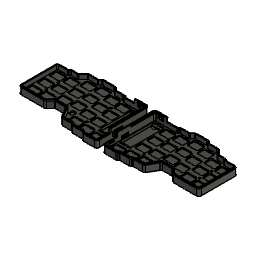
mriya-classic-fdm-301645-v1.00 (Autodesk Fusion 360 design; units mm, degrees)
Autodesk Fusion 360 part; units mm, degrees
(part 1 of 2)
sketch "mriya-classic-fdm-301645" plane through (0, 0, 0) normal (0, 0, 1) x (1, 0, 0)
  line L0 (-101.0213, 15.6719) -> (-94.7787, 21.9145) construction
  line L1 (-26.4858, 1.079) -> (-27.6142, 2.2074) construction
  line L2 (-138.1, 14.7932) -> (-103.1426, 14.7932) construction
  line L3 (-44.0716, 2.7932) -> (-29.0284, 2.7932) construction
  line L4 (-8.6, 0.4932) -> (-25.0716, 0.4932) construction
  line L5 (-64.4741, 6.1094) -> (-72.7517, 20.7608) construction
  line L6 (-45.4858, 3.379) -> (-46.6142, 4.5074) construction
  line L7 (-122.6142, 71.579) -> (-121.4858, 72.7074) construction
  line L8 (-101.0716, 81.2932) -> (-87.2284, 81.2932) construction
  line L9 (-138.1, 70.9932) -> (-124.0284, 70.9932) construction
  line L10 (-92.6574, 22.7932) -> (-76.2344, 22.7932) construction
  line L11 (-48.0284, 5.0932) -> (-62.7328, 5.0932) construction
  line L12 (-82.0716, 84.7932) -> (-64.7284, 84.7932) construction
  line L13 (-58.5716, 80.2932) -> (-45.7284, 80.2932) construction
  line L14 (-24.1, 19.4932) -> (-7.1, 19.4932) construction
  line L15 (-25.6, 20.9932) -> (-25.6, 77.9932) construction
  line L16 (-83.4858, 84.2074) -> (-85.8142, 81.879) construction
  line L17 (-63.3142, 84.2074) -> (-59.9858, 80.879) construction
  line L18 (-139.6, 69.4932) -> (-139.6, 16.2932) construction
  line L19 (-43.1858, 78.579) -> (-44.3142, 79.7074) construction
  line L20 (-99.4, 40.3932) -> (-99.4, 27.9932) construction
  line L21 (-98.6, 41.1932) -> (-86.2, 41.1932) construction
  line L22 (-98.6, 27.1932) -> (-86.2, 27.1932) construction
  line L23 (-85.4, 40.3932) -> (-85.4, 27.9932) construction
  line L24 (-42.4, 56.0932) -> (-42.4, 43.6932) construction
  line L25 (-41.6, 56.8932) -> (-29.2, 56.8932) construction
  line L26 (-41.6, 42.8932) -> (-29.2, 42.8932) construction
  line L27 (-28.4, 56.0932) -> (-28.4, 43.6932) construction
  line L28 (-61.4, 58.3932) -> (-61.4, 45.9932) construction
  line L29 (-60.6, 59.1932) -> (-48.2, 59.1932) construction
  line L30 (-60.6, 45.1932) -> (-48.2, 45.1932) construction
  line L31 (-47.4, 58.3932) -> (-47.4, 45.9932) construction
  line L32 (-137.4, 68.0932) -> (-137.4, 55.6932) construction
  line L33 (-136.6, 68.8932) -> (-124.2, 68.8932) construction
  line L34 (-136.6, 54.8932) -> (-124.2, 54.8932) construction
  line L35 (-123.4, 68.0932) -> (-123.4, 55.6932) construction
  line L36 (-61.4, 39.3932) -> (-61.4, 26.9932) construction
  line L37 (-60.6, 40.1932) -> (-48.2, 40.1932) construction
  line L38 (-60.6, 26.1932) -> (-48.2, 26.1932) construction
  line L39 (-47.4, 39.3932) -> (-47.4, 26.9932) construction
  line L40 (-42.4, 18.0932) -> (-42.4, 5.6932) construction
  line L41 (-41.6, 18.8932) -> (-29.2, 18.8932) construction
  line L42 (-41.6, 4.8932) -> (-29.2, 4.8932) construction
  line L43 (-28.4, 18.0932) -> (-28.4, 5.6932) construction
  line L44 (-23.4, 15.7932) -> (-23.4, 3.3932) construction
  line L45 (-22.6, 16.5932) -> (-10.2, 16.5932) construction
  line L46 (-22.6, 2.5932) -> (-10.2, 2.5932) construction
  line L47 (-9.4, 15.7932) -> (-9.4, 3.3932) construction
  line L48 (-137.4, 49.0932) -> (-137.4, 36.6932) construction
  line L49 (-136.6, 49.8932) -> (-124.2, 49.8932) construction
  line L50 (-136.6, 35.8932) -> (-124.2, 35.8932) construction
  line L51 (-123.4, 49.0932) -> (-123.4, 36.6932) construction
  line L52 (-118.4, 51.3932) -> (-118.4, 38.9932) construction
  line L53 (-117.6, 52.1932) -> (-105.2, 52.1932) construction
  line L54 (-117.6, 38.1932) -> (-105.2, 38.1932) construction
  line L55 (-104.4, 51.3932) -> (-104.4, 38.9932) construction
  line L56 (-137.4, 30.0932) -> (-137.4, 17.6932) construction
  line L57 (-136.6, 30.8932) -> (-124.2, 30.8932) construction
  line L58 (-136.6, 16.8932) -> (-124.2, 16.8932) construction
  line L59 (-123.4, 30.0932) -> (-123.4, 17.6932) construction
  line L60 (-61.4, 20.3932) -> (-61.4, 7.9932) construction
  line L61 (-60.6, 21.1932) -> (-48.2, 21.1932) construction
  line L62 (-60.6, 7.1932) -> (-48.2, 7.1932) construction
  line L63 (-47.4, 20.3932) -> (-47.4, 7.9932) construction
  line L64 (-80.4, 43.8932) -> (-80.4, 31.4932) construction
  line L65 (-79.6, 44.6932) -> (-67.2, 44.6932) construction
  line L66 (-79.6, 30.6932) -> (-67.2, 30.6932) construction
  line L67 (-66.4, 43.8932) -> (-66.4, 31.4932) construction
  line L68 (-80.4, 81.8932) -> (-80.4, 69.4932) construction
  line L69 (-79.6, 82.6932) -> (-67.2, 82.6932) construction
  line L70 (-79.6, 68.6932) -> (-67.2, 68.6932) construction
  line L71 (-66.4, 81.8932) -> (-66.4, 69.4932) construction
  line L72 (-42.4, 37.0932) -> (-42.4, 24.6932) construction
  line L73 (-41.6, 37.8932) -> (-29.2, 37.8932) construction
  line L74 (-41.6, 23.8932) -> (-29.2, 23.8932) construction
  line L75 (-28.4, 37.0932) -> (-28.4, 24.6932) construction
  line L76 (-118.4, 32.3932) -> (-118.4, 19.9932) construction
  line L77 (-117.6, 33.1932) -> (-105.2, 33.1932) construction
  line L78 (-117.6, 19.1932) -> (-105.2, 19.1932) construction
  line L79 (-104.4, 32.3932) -> (-104.4, 19.9932) construction
  line L80 (-61.4, 77.3932) -> (-61.4, 64.9932) construction
  line L81 (-60.6, 78.1932) -> (-48.2, 78.1932) construction
  line L82 (-60.6, 64.1932) -> (-48.2, 64.1932) construction
  line L83 (-47.4, 77.3932) -> (-47.4, 64.9932) construction
  line L84 (-42.4, 75.0932) -> (-42.4, 62.6932) construction
  line L85 (-41.6, 75.8932) -> (-29.2, 75.8932) construction
  line L86 (-41.6, 61.8932) -> (-29.2, 61.8932) construction
  line L87 (-28.4, 75.0932) -> (-28.4, 62.6932) construction
  line L88 (-118.4, 70.3932) -> (-118.4, 57.9932) construction
  line L89 (-117.6, 71.1932) -> (-105.2, 71.1932) construction
  line L90 (-117.6, 57.1932) -> (-105.2, 57.1932) construction
  line L91 (-104.4, 70.3932) -> (-104.4, 57.9932) construction
  line L92 (-99.4, 59.3932) -> (-99.4, 46.9932) construction
  line L93 (-98.6, 60.1932) -> (-86.2, 60.1932) construction
  line L94 (-98.6, 46.1932) -> (-86.2, 46.1932) construction
  line L95 (-85.4, 59.3932) -> (-85.4, 46.9932) construction
  line L96 (-80.4, 62.8932) -> (-80.4, 50.4932) construction
  line L97 (-79.6, 63.6932) -> (-67.2, 63.6932) construction
  line L98 (-79.6, 49.6932) -> (-67.2, 49.6932) construction
  line L99 (-66.4, 62.8932) -> (-66.4, 50.4932) construction
  line L100 (-99.4, 78.3932) -> (-99.4, 65.9932) construction
  line L101 (-98.6, 79.1932) -> (-86.2, 79.1932) construction
  line L102 (-98.6, 65.1932) -> (-86.2, 65.1932) construction
  line L103 (-85.4, 78.3932) -> (-85.4, 65.9932) construction
  circle A0 centre (-120.9, 53.5432) radius 1.7
  circle A1 centre (-120.9, 34.5432) radius 1.7
  circle A2 centre (-68.3, 23.4932) radius 4
  circle A3 centre (-44.9, 22.5432) radius 1.7
  circle A4 centre (-44.9, 60.5432) radius 1.7
  arc A5 (-43.1858, 78.579) -> (-41.7716, 77.9932) centre (-41.7716, 79.9932) ccw construction
  arc A6 (-44.3142, 79.7074) -> (-45.7284, 80.2932) centre (-45.7285, 78.2931) ccw construction
  arc A7 (-59.9858, 80.879) -> (-58.5716, 80.2932) centre (-58.5716, 82.2931) ccw construction
  arc A8 (-63.3142, 84.2074) -> (-64.7284, 84.7932) centre (-64.7285, 82.7931) ccw construction
  arc A9 (-82.0716, 84.7932) -> (-83.4858, 84.2074) centre (-82.0716, 82.7933) ccw construction
  arc A10 (-87.2284, 81.2932) -> (-85.8142, 81.879) centre (-87.2284, 83.2932) ccw construction
  arc A11 (-101.0716, 81.2932) -> (-102.4858, 80.7074) centre (-101.0716, 79.2933) ccw construction
  arc A12 (-120.0716, 73.2932) -> (-121.4858, 72.7074) centre (-120.0716, 71.2933) ccw construction
  arc A13 (-124.0284, 70.9932) -> (-122.6142, 71.579) centre (-124.0284, 72.9932) ccw construction
  arc A14 (-138.1, 70.9932) -> (-139.6, 69.4932) centre (-138.1, 69.4932) ccw construction
  arc A15 (-139.6, 16.2932) -> (-138.1, 14.7932) centre (-138.1, 16.2932) ccw construction
  arc A16 (-103.1426, 14.7932) -> (-101.0213, 15.6719) centre (-103.1426, 17.7931) ccw construction
  arc A17 (-92.6574, 22.7932) -> (-94.7787, 21.9145) centre (-92.6573, 19.7931) ccw construction
  arc A18 (-72.7517, 20.7608) -> (-76.2344, 22.7932) centre (-76.2344, 18.793) ccw construction
  arc A19 (-64.4741, 6.1094) -> (-62.7328, 5.0932) centre (-62.7328, 7.0932) ccw construction
  arc A20 (-46.6142, 4.5074) -> (-48.0284, 5.0932) centre (-48.0284, 3.0933) ccw construction
  arc A21 (-45.4858, 3.379) -> (-44.0716, 2.7932) centre (-44.0715, 4.7933) ccw construction
  arc A22 (-27.6142, 2.2074) -> (-29.0284, 2.7932) centre (-29.0284, 0.7933) ccw construction
  arc A23 (-26.4858, 1.079) -> (-25.0716, 0.4932) centre (-25.0715, 2.4933) ccw construction
  arc A24 (-8.6, 0.4932) -> (-7.1, 1.9932) centre (-8.6, 1.9932) ccw construction
  arc A25 (-25.6, 20.9932) -> (-24.1, 19.4932) centre (-24.1, 20.9932) ccw construction
  line L104 (-7.1, 1.9932) -> (-7.1, 76.4932) construction
  line L105 (-41.7716, 77.9932) -> (-8.6, 77.9932) construction
  arc A26 (-7.1, 76.4932) -> (-8.6, 77.9932) centre (-8.6, 76.4932) ccw construction
  arc A27 (-136.6, 68.8932) -> (-137.4, 68.0932) centre (-136.6, 68.0932) ccw construction
  arc A28 (-123.4, 68.0932) -> (-124.2, 68.8932) centre (-124.2, 68.0932) ccw construction
  arc A29 (-124.2, 54.8932) -> (-123.4, 55.6932) centre (-124.2, 55.6932) ccw construction
  arc A30 (-137.4, 55.6932) -> (-136.6, 54.8932) centre (-136.6, 55.6932) ccw construction
  arc A31 (-136.6, 49.8932) -> (-137.4, 49.0932) centre (-136.6, 49.0932) ccw construction
  arc A32 (-123.4, 49.0932) -> (-124.2, 49.8932) centre (-124.2, 49.0932) ccw construction
  arc A33 (-124.2, 35.8932) -> (-123.4, 36.6932) centre (-124.2, 36.6932) ccw construction
  arc A34 (-137.4, 36.6932) -> (-136.6, 35.8932) centre (-136.6, 36.6932) ccw construction
  arc A35 (-136.6, 30.8932) -> (-137.4, 30.0932) centre (-136.6, 30.0932) ccw construction
  arc A36 (-123.4, 30.0932) -> (-124.2, 30.8932) centre (-124.2, 30.0932) ccw construction
  arc A37 (-124.2, 16.8932) -> (-123.4, 17.6932) centre (-124.2, 17.6932) ccw construction
  arc A38 (-137.4, 17.6932) -> (-136.6, 16.8932) centre (-136.6, 17.6932) ccw construction
  arc A39 (-118.4, 19.9932) -> (-117.6, 19.1932) centre (-117.6, 19.9932) ccw construction
  arc A40 (-105.2, 19.1932) -> (-104.4, 19.9932) centre (-105.2, 19.9932) ccw construction
  arc A41 (-104.4, 32.3932) -> (-105.2, 33.1932) centre (-105.2, 32.3932) ccw construction
  arc A42 (-117.6, 33.1932) -> (-118.4, 32.3932) centre (-117.6, 32.3932) ccw construction
  arc A43 (-105.2, 38.1932) -> (-104.4, 38.9932) centre (-105.2, 38.9932) ccw construction
  arc A44 (-118.4, 38.9932) -> (-117.6, 38.1932) centre (-117.6, 38.9932) ccw construction
  arc A45 (-117.6, 52.1932) -> (-118.4, 51.3932) centre (-117.6, 51.3932) ccw construction
  arc A46 (-104.4, 51.3932) -> (-105.2, 52.1932) centre (-105.2, 51.3932) ccw construction
  arc A47 (-118.4, 57.9932) -> (-117.6, 57.1932) centre (-117.6, 57.9932) ccw construction
  arc A48 (-105.2, 57.1932) -> (-104.4, 57.9932) centre (-105.2, 57.9932) ccw construction
  arc A49 (-104.4, 70.3932) -> (-105.2, 71.1932) centre (-105.2, 70.3932) ccw construction
  arc A50 (-117.6, 71.1932) -> (-118.4, 70.3932) centre (-117.6, 70.3932) ccw construction
  arc A51 (-98.6, 79.1932) -> (-99.4, 78.3932) centre (-98.6, 78.3932) ccw construction
  arc A52 (-85.4, 78.3932) -> (-86.2, 79.1932) centre (-86.2, 78.3932) ccw construction
  arc A53 (-86.2, 65.1932) -> (-85.4, 65.9932) centre (-86.2, 65.9932) ccw construction
  arc A54 (-99.4, 65.9932) -> (-98.6, 65.1932) centre (-98.6, 65.9932) ccw construction
  arc A55 (-98.6, 60.1932) -> (-99.4, 59.3932) centre (-98.6, 59.3932) ccw construction
  arc A56 (-85.4, 59.3932) -> (-86.2, 60.1932) centre (-86.2, 59.3932) ccw construction
  arc A57 (-86.2, 46.1932) -> (-85.4, 46.9932) centre (-86.2, 46.9932) ccw construction
  arc A58 (-99.4, 46.9932) -> (-98.6, 46.1932) centre (-98.6, 46.9932) ccw construction
  arc A59 (-98.6, 41.1932) -> (-99.4, 40.3932) centre (-98.6, 40.3932) ccw construction
  arc A60 (-99.4, 27.9932) -> (-98.6, 27.1932) centre (-98.6, 27.9932) ccw construction
  arc A61 (-86.2, 27.1932) -> (-85.4, 27.9932) centre (-86.2, 27.9932) ccw construction
  arc A62 (-85.4, 40.3932) -> (-86.2, 41.1932) centre (-86.2, 40.3932) ccw construction
  arc A63 (-80.4, 31.4932) -> (-79.6, 30.6932) centre (-79.6, 31.4932) ccw construction
  arc A64 (-79.6, 44.6932) -> (-80.4, 43.8932) centre (-79.6, 43.8932) ccw construction
  arc A65 (-66.4, 43.8932) -> (-67.2, 44.6932) centre (-67.2, 43.8932) ccw construction
  arc A66 (-67.2, 30.6932) -> (-66.4, 31.4932) centre (-67.2, 31.4932) ccw construction
  arc A67 (-67.2, 49.6932) -> (-66.4, 50.4932) centre (-67.2, 50.4932) ccw construction
  arc A68 (-80.4, 50.4932) -> (-79.6, 49.6932) centre (-79.6, 50.4932) ccw construction
  arc A69 (-79.6, 63.6932) -> (-80.4, 62.8932) centre (-79.6, 62.8932) ccw construction
  arc A70 (-66.4, 62.8932) -> (-67.2, 63.6932) centre (-67.2, 62.8932) ccw construction
  arc A71 (-67.2, 68.6932) -> (-66.4, 69.4932) centre (-67.2, 69.4932) ccw construction
  arc A72 (-80.4, 69.4932) -> (-79.6, 68.6932) centre (-79.6, 69.4932) ccw construction
  arc A73 (-79.6, 82.6932) -> (-80.4, 81.8932) centre (-79.6, 81.8932) ccw construction
  arc A74 (-66.4, 81.8932) -> (-67.2, 82.6932) centre (-67.2, 81.8932) ccw construction
  arc A75 (-60.6, 78.1932) -> (-61.4, 77.3932) centre (-60.6, 77.3932) ccw construction
  arc A76 (-61.4, 64.9932) -> (-60.6, 64.1932) centre (-60.6, 64.9932) ccw construction
  arc A77 (-48.2, 64.1932) -> (-47.4, 64.9932) centre (-48.2, 64.9932) ccw construction
  arc A78 (-47.4, 77.3932) -> (-48.2, 78.1932) centre (-48.2, 77.3932) ccw construction
  arc A79 (-47.4, 58.3932) -> (-48.2, 59.1932) centre (-48.2, 58.3932) ccw construction
  arc A80 (-60.6, 59.1932) -> (-61.4, 58.3932) centre (-60.6, 58.3932) ccw construction
  arc A81 (-61.4, 45.9932) -> (-60.6, 45.1932) centre (-60.6, 45.9932) ccw construction
  arc A82 (-48.2, 45.1932) -> (-47.4, 45.9932) centre (-48.2, 45.9932) ccw construction
  arc A83 (-47.4, 39.3932) -> (-48.2, 40.1932) centre (-48.2, 39.3932) ccw construction
  arc A84 (-60.6, 40.1932) -> (-61.4, 39.3932) centre (-60.6, 39.3932) ccw construction
  arc A85 (-61.4, 26.9932) -> (-60.6, 26.1932) centre (-60.6, 26.9932) ccw construction
  arc A86 (-48.2, 26.1932) -> (-47.4, 26.9932) centre (-48.2, 26.9932) ccw construction
  arc A87 (-47.4, 20.3932) -> (-48.2, 21.1932) centre (-48.2, 20.3932) ccw construction
  arc A88 (-60.6, 21.1932) -> (-61.4, 20.3932) centre (-60.6, 20.3932) ccw construction
  arc A89 (-61.4, 7.9932) -> (-60.6, 7.1932) centre (-60.6, 7.9932) ccw construction
  arc A90 (-48.2, 7.1932) -> (-47.4, 7.9932) centre (-48.2, 7.9932) ccw construction
  arc A91 (-42.4, 5.6932) -> (-41.6, 4.8932) centre (-41.6, 5.6932) ccw construction
  arc A92 (-29.2, 4.8932) -> (-28.4, 5.6932) centre (-29.2, 5.6932) ccw construction
  arc A93 (-28.4, 18.0932) -> (-29.2, 18.8932) centre (-29.2, 18.0932) ccw construction
  arc A94 (-41.6, 18.8932) -> (-42.4, 18.0932) centre (-41.6, 18.0932) ccw construction
  arc A95 (-23.4, 3.3932) -> (-22.6, 2.5932) centre (-22.6, 3.3932) ccw construction
  arc A96 (-10.2, 2.5932) -> (-9.4, 3.3932) centre (-10.2, 3.3932) ccw construction
  arc A97 (-9.4, 15.7932) -> (-10.2, 16.5932) centre (-10.2, 15.7932) ccw construction
  arc A98 (-22.6, 16.5932) -> (-23.4, 15.7932) centre (-22.6, 15.7932) ccw construction
  arc A99 (-29.2, 23.8932) -> (-28.4, 24.6932) centre (-29.2, 24.6932) ccw construction
  arc A100 (-42.4, 24.6932) -> (-41.6, 23.8932) centre (-41.6, 24.6932) ccw construction
  arc A101 (-41.6, 37.8932) -> (-42.4, 37.0932) centre (-41.6, 37.0932) ccw construction
  arc A102 (-28.4, 37.0932) -> (-29.2, 37.8932) centre (-29.2, 37.0932) ccw construction
  arc A103 (-29.2, 42.8932) -> (-28.4, 43.6932) centre (-29.2, 43.6932) ccw construction
  arc A104 (-42.4, 43.6932) -> (-41.6, 42.8932) centre (-41.6, 43.6932) ccw construction
  arc A105 (-41.6, 56.8932) -> (-42.4, 56.0932) centre (-41.6, 56.0932) ccw construction
  arc A106 (-28.4, 56.0932) -> (-29.2, 56.8932) centre (-29.2, 56.0932) ccw construction
  arc A107 (-29.2, 61.8932) -> (-28.4, 62.6932) centre (-29.2, 62.6932) ccw construction
  arc A108 (-42.4, 62.6932) -> (-41.6, 61.8932) centre (-41.6, 62.6932) ccw construction
  arc A109 (-41.6, 75.8932) -> (-42.4, 75.0932) centre (-41.6, 75.0932) ccw construction
  arc A110 (-28.4, 75.0932) -> (-29.2, 75.8932) centre (-29.2, 75.0932) ccw construction
  circle A111 centre (-22.6, 22.4932) radius 1.15
  circle A112 centre (-10.1, 22.4932) radius 1.15
  line L106 (-102.4858, 80.7074) -> (-109.0213, 74.1719) construction
  line L107 (-120.0716, 73.2932) -> (-111.1426, 73.2932) construction
  arc A113 (-111.1426, 73.2932) -> (-109.0213, 74.1719) centre (-111.1426, 76.2932) ccw construction
  arc A114 (-64.7284, 82.7932) -> (-64.7285, 82.7932) centre (-64.7285, 82.7931) ccw
  arc A115 (-45.7284, 78.2932) -> (-45.7285, 78.2932) centre (-45.7285, 78.2931) ccw
  arc A116 (-25.0716, 2.4932) -> (-25.0715, 2.4932) centre (-25.0715, 2.4933) ccw
  arc A117 (-44.0716, 4.7932) -> (-44.0715, 4.7932) centre (-44.0715, 4.7933) ccw
  line L108 (-138.9, 58.3932) -> (-138.9, 66.8932)
  line L109 (-136.9, 68.8932) -> (-123.9, 68.8932)
  arc A118 (-121.9, 66.8932) -> (-123.9, 68.8932) centre (-123.9, 66.8932) ccw
  arc A119 (-138.9, 58.3932) -> (-136.9, 56.3932) centre (-136.9, 58.3932) ccw
  arc A120 (-136.9, 68.8932) -> (-138.9, 66.8932) centre (-136.9, 66.8932) ccw
  arc A121 (-138.9, 39.3932) -> (-136.9, 37.3932) centre (-136.9, 39.3932) ccw
  line L110 (-138.9, 39.3932) -> (-138.9, 47.8932)
  arc A122 (-136.9, 49.8932) -> (-138.9, 47.8932) centre (-136.9, 47.8932) ccw
  line L111 (-136.9, 49.8932) -> (-123.9, 49.8932)
  arc A123 (-121.9, 47.8932) -> (-123.9, 49.8932) centre (-123.9, 47.8932) ccw
  arc A124 (-123.9, 18.3932) -> (-121.9, 20.3932) centre (-123.9, 20.3932) ccw
  line L112 (-123.9, 18.3932) -> (-136.9, 18.3932)
  arc A125 (-138.9, 20.3932) -> (-136.9, 18.3932) centre (-136.9, 20.3932) ccw
  line L113 (-138.9, 20.3932) -> (-138.9, 28.8932)
  arc A126 (-136.9, 30.8932) -> (-138.9, 28.8932) centre (-136.9, 28.8932) ccw
  line L114 (-136.9, 30.8932) -> (-123.9, 30.8932)
  arc A127 (-121.9, 28.8932) -> (-123.9, 30.8932) centre (-123.9, 28.8932) ccw
  line L115 (-121.9, 28.8932) -> (-121.9, 20.3932)
  arc A128 (-104.9, 58.6932) -> (-102.9, 60.6932) centre (-104.9, 60.6932) ccw
  line L116 (-104.9, 58.6932) -> (-117.9, 58.6932)
  arc A129 (-119.9, 60.6932) -> (-117.9, 58.6932) centre (-117.9, 60.6932) ccw
  line L117 (-119.9, 60.6932) -> (-119.9, 69.1932)
  arc A130 (-117.9, 71.1932) -> (-119.9, 69.1932) centre (-117.9, 69.1932) ccw
  line L118 (-117.9, 71.1932) -> (-104.9, 71.1932)
  arc A131 (-102.9, 69.1932) -> (-104.9, 71.1932) centre (-104.9, 69.1932) ccw
  line L119 (-102.9, 69.1932) -> (-102.9, 60.6932)
  arc A132 (-104.9, 39.6932) -> (-102.9, 41.6932) centre (-104.9, 41.6932) ccw
  line L120 (-104.9, 39.6932) -> (-117.9, 39.6932)
  arc A133 (-119.9, 41.6932) -> (-117.9, 39.6932) centre (-117.9, 41.6932) ccw
  arc A134 (-102.9, 50.1932) -> (-104.9, 52.1932) centre (-104.9, 50.1932) ccw
  line L121 (-102.9, 50.1932) -> (-102.9, 41.6932)
  arc A135 (-104.9, 20.6932) -> (-102.9, 22.6932) centre (-104.9, 22.6932) ccw
  line L122 (-104.9, 20.6932) -> (-117.9, 20.6932)
  arc A136 (-119.9, 22.6932) -> (-117.9, 20.6932) centre (-117.9, 22.6932) ccw
  arc A137 (-102.9, 31.1932) -> (-104.9, 33.1932) centre (-104.9, 31.1932) ccw
  line L123 (-102.9, 31.1932) -> (-102.9, 22.6932)
  arc A138 (-85.9, 66.6932) -> (-83.9, 68.6932) centre (-85.9, 68.6932) ccw
  line L124 (-85.9, 66.6932) -> (-98.9, 66.6932)
  arc A139 (-100.9, 68.6932) -> (-98.9, 66.6932) centre (-98.9, 68.6932) ccw
  line L125 (-100.9, 68.6932) -> (-100.9, 77.1932)
  arc A140 (-98.9, 79.1932) -> (-100.9, 77.1932) centre (-98.9, 77.1932) ccw
  line L126 (-98.9, 79.1932) -> (-85.9, 79.1932)
  arc A141 (-83.9, 77.1932) -> (-85.9, 79.1932) centre (-85.9, 77.1932) ccw
  line L127 (-83.9, 77.1932) -> (-83.9, 68.6932)
  arc A142 (-85.9, 47.6932) -> (-83.9, 49.6932) centre (-85.9, 49.6932) ccw
  line L128 (-85.9, 47.6932) -> (-98.9, 47.6932)
  arc A143 (-100.9, 49.6932) -> (-98.9, 47.6932) centre (-98.9, 49.6932) ccw
  line L129 (-100.9, 49.6932) -> (-100.9, 58.1932)
  arc A144 (-98.9, 60.1932) -> (-100.9, 58.1932) centre (-98.9, 58.1932) ccw
  line L130 (-98.9, 60.1932) -> (-85.9, 60.1932)
  arc A145 (-83.9, 58.1932) -> (-85.9, 60.1932) centre (-85.9, 58.1932) ccw
  line L131 (-83.9, 58.1932) -> (-83.9, 49.6932)
  arc A146 (-85.9, 28.6932) -> (-83.9, 30.6932) centre (-85.9, 30.6932) ccw
  line L132 (-85.9, 28.6932) -> (-98.9, 28.6932)
  arc A147 (-100.9, 30.6932) -> (-98.9, 28.6932) centre (-98.9, 30.6932) ccw
  line L133 (-100.9, 30.6932) -> (-100.9, 39.1932)
  arc A148 (-98.9, 41.1932) -> (-100.9, 39.1932) centre (-98.9, 39.1932) ccw
  line L134 (-98.9, 41.1932) -> (-85.9, 41.1932)
  arc A149 (-83.9, 39.1932) -> (-85.9, 41.1932) centre (-85.9, 39.1932) ccw
  line L135 (-83.9, 39.1932) -> (-83.9, 30.6932)
  arc A150 (-66.9, 32.1932) -> (-64.9, 34.1932) centre (-66.9, 34.1932) ccw
  line L136 (-66.9, 32.1932) -> (-79.9, 32.1932)
  arc A151 (-81.9, 34.1932) -> (-79.9, 32.1932) centre (-79.9, 34.1932) ccw
  line L137 (-81.9, 34.1932) -> (-81.9, 42.6932)
  arc A152 (-79.9, 44.6932) -> (-81.9, 42.6932) centre (-79.9, 42.6932) ccw
  line L138 (-79.9, 44.6932) -> (-66.9, 44.6932)
  arc A153 (-64.9, 42.6932) -> (-66.9, 44.6932) centre (-66.9, 42.6932) ccw
  line L139 (-64.9, 42.6932) -> (-64.9, 34.1932)
  arc A154 (-66.9, 51.1932) -> (-64.9, 53.1932) centre (-66.9, 53.1932) ccw
  line L140 (-66.9, 51.1932) -> (-79.9, 51.1932)
  arc A155 (-81.9, 53.1932) -> (-79.9, 51.1932) centre (-79.9, 53.1932) ccw
  line L141 (-81.9, 53.1932) -> (-81.9, 61.6932)
  arc A156 (-79.9, 63.6932) -> (-81.9, 61.6932) centre (-79.9, 61.6932) ccw
  line L142 (-79.9, 63.6932) -> (-66.9, 63.6932)
  arc A157 (-64.9, 61.6932) -> (-66.9, 63.6932) centre (-66.9, 61.6932) ccw
  line L143 (-64.9, 61.6932) -> (-64.9, 53.1932)
  arc A158 (-66.9, 70.1932) -> (-64.9, 72.1932) centre (-66.9, 72.1932) ccw
  line L144 (-66.9, 70.1932) -> (-79.9, 70.1932)
  arc A159 (-81.9, 72.1932) -> (-79.9, 70.1932) centre (-79.9, 72.1932) ccw
  line L145 (-81.9, 72.1932) -> (-81.9, 80.6932)
  arc A160 (-79.9, 82.6932) -> (-81.9, 80.6932) centre (-79.9, 80.6932) ccw
  line L146 (-79.9, 82.6932) -> (-66.9, 82.6932)
  arc A161 (-64.9, 80.6932) -> (-66.9, 82.6932) centre (-66.9, 80.6932) ccw
  line L147 (-64.9, 80.6932) -> (-64.9, 72.1932)
  arc A162 (-47.9, 27.6932) -> (-45.9, 29.6932) centre (-47.9, 29.6932) ccw
  line L148 (-47.9, 27.6932) -> (-60.9, 27.6932)
  arc A163 (-62.9, 29.6932) -> (-60.9, 27.6932) centre (-60.9, 29.6932) ccw
  line L149 (-62.9, 29.6932) -> (-62.9, 38.1932)
  arc A164 (-60.9, 40.1932) -> (-62.9, 38.1932) centre (-60.9, 38.1932) ccw
  line L150 (-60.9, 40.1932) -> (-47.9, 40.1932)
  arc A165 (-45.9, 38.1932) -> (-47.9, 40.1932) centre (-47.9, 38.1932) ccw
  line L151 (-45.9, 38.1932) -> (-45.9, 29.6932)
  arc A166 (-47.9, 46.6932) -> (-45.9, 48.6932) centre (-47.9, 48.6932) ccw
  line L152 (-47.9, 46.6932) -> (-60.9, 46.6932)
  arc A167 (-62.9, 48.6932) -> (-60.9, 46.6932) centre (-60.9, 48.6932) ccw
  line L153 (-62.9, 48.6932) -> (-62.9, 57.1932)
  arc A168 (-60.9, 59.1932) -> (-62.9, 57.1932) centre (-60.9, 57.1932) ccw
  arc A169 (-47.9, 65.6932) -> (-45.9, 67.6932) centre (-47.9, 67.6932) ccw
  line L154 (-47.9, 65.6932) -> (-60.9, 65.6932)
  arc A170 (-62.9, 67.6932) -> (-60.9, 65.6932) centre (-60.9, 67.6932) ccw
  line L155 (-62.9, 67.6932) -> (-62.9, 76.1932)
  arc A171 (-60.9, 78.1932) -> (-62.9, 76.1932) centre (-60.9, 76.1932) ccw
  line L156 (-60.9, 78.1932) -> (-47.9, 78.1932)
  arc A172 (-45.9, 76.1932) -> (-47.9, 78.1932) centre (-47.9, 76.1932) ccw
  line L157 (-45.9, 76.1932) -> (-45.9, 67.6932)
  arc A173 (-47.9, 8.6932) -> (-45.9, 10.6932) centre (-47.9, 10.6932) ccw
  line L158 (-47.9, 8.6932) -> (-60.9, 8.6932)
  arc A174 (-62.9, 10.6932) -> (-60.9, 8.6932) centre (-60.9, 10.6932) ccw
  line L159 (-62.9, 10.6932) -> (-62.9, 19.1932)
  arc A175 (-60.9, 21.1932) -> (-62.9, 19.1932) centre (-60.9, 19.1932) ccw
  arc A176 (-28.9, 6.3932) -> (-26.9, 8.3932) centre (-28.9, 8.3932) ccw
  line L160 (-28.9, 6.3932) -> (-41.9, 6.3932)
  arc A177 (-43.9, 8.3932) -> (-41.9, 6.3932) centre (-41.9, 8.3932) ccw
  line L161 (-43.9, 8.3932) -> (-43.9, 16.8932)
  arc A178 (-41.9, 18.8932) -> (-43.9, 16.8932) centre (-41.9, 16.8932) ccw
  line L162 (-41.9, 18.8932) -> (-28.9, 18.8932)
  arc A179 (-26.9, 16.8932) -> (-28.9, 18.8932) centre (-28.9, 16.8932) ccw
  line L163 (-26.9, 16.8932) -> (-26.9, 8.3932)
  arc A180 (-28.9, 25.3932) -> (-26.9, 27.3932) centre (-28.9, 27.3932) ccw
  arc A181 (-41.9, 37.8932) -> (-43.9, 35.8932) centre (-41.9, 35.8932) ccw
  line L164 (-41.9, 37.8932) -> (-28.9, 37.8932)
  arc A182 (-26.9, 35.8932) -> (-28.9, 37.8932) centre (-28.9, 35.8932) ccw
  line L165 (-26.9, 35.8932) -> (-26.9, 27.3932)
  arc A183 (-28.9, 44.3932) -> (-26.9, 46.3932) centre (-28.9, 46.3932) ccw
  line L166 (-28.9, 44.3932) -> (-41.9, 44.3932)
  arc A184 (-43.9, 46.3932) -> (-41.9, 44.3932) centre (-41.9, 46.3932) ccw
  line L167 (-43.9, 46.3932) -> (-43.9, 54.8932)
  arc A185 (-41.9, 56.8932) -> (-43.9, 54.8932) centre (-41.9, 54.8932) ccw
  line L168 (-41.9, 56.8932) -> (-28.9, 56.8932)
  arc A186 (-26.9, 54.8932) -> (-28.9, 56.8932) centre (-28.9, 54.8932) ccw
  line L169 (-26.9, 54.8932) -> (-26.9, 46.3932)
  arc A187 (-28.9, 63.3932) -> (-26.9, 65.3932) centre (-28.9, 65.3932) ccw
  arc A188 (-41.9, 75.8932) -> (-43.9, 73.8932) centre (-41.9, 73.8932) ccw
  line L170 (-41.9, 75.8932) -> (-28.9, 75.8932)
  arc A189 (-26.9, 73.8932) -> (-28.9, 75.8932) centre (-28.9, 73.8932) ccw
  line L171 (-26.9, 73.8932) -> (-26.9, 65.3932)
  arc A190 (-9.7, 4.0932) -> (-7.7, 6.0932) centre (-9.7, 6.0932) ccw
  line L172 (-9.7, 4.0932) -> (-23, 4.0932)
  arc A191 (-25, 6.0932) -> (-23, 4.0932) centre (-23, 6.0932) ccw
  line L173 (-25, 6.0932) -> (-25, 14.5932)
  arc A192 (-23, 16.5932) -> (-25, 14.5932) centre (-23, 14.5932) ccw
  line L174 (-23, 16.5932) -> (-9.7, 16.5932)
  arc A193 (-7.7, 14.5932) -> (-9.7, 16.5932) centre (-9.7, 14.5932) ccw
  line L175 (-7.7, 14.5932) -> (-7.7, 6.0932)
  line L176 (-25.8, 78.1932) -> (-25.8, 80.6932)
  line L177 (-6.9, 19.2932) -> (-4.4, 19.2932)
  line L178 (-121.9, 47.8932) -> (-121.9, 39.3932)
  line L179 (-123.9, 37.3932) -> (-136.9, 37.3932)
  line L180 (-117.4787, 33.1932) -> (-104.9, 33.1932)
  line L181 (-119.9, 22.6932) -> (-119.9, 30.7719)
  line L182 (-118.5393, 32.7539) -> (-119.4607, 31.8325)
  line L183 (-121.9, 66.8932) -> (-121.9, 58.3932)
  line L184 (-123.9, 56.3932) -> (-136.9, 56.3932)
  line L185 (-117.4787, 52.1932) -> (-104.9, 52.1932)
  line L186 (-119.9, 41.6932) -> (-119.9, 49.7719)
  line L187 (-118.5393, 51.7539) -> (-119.4607, 50.8325)
  arc A194 (-117.4787, 52.1932) -> (-118.5393, 51.7539) centre (-117.4787, 50.6932) ccw
  arc A195 (-119.4607, 50.8325) -> (-119.9, 49.7719) centre (-118.4, 49.7719) ccw
  arc A196 (-119.4607, 31.8325) -> (-119.9, 30.7719) centre (-118.4, 30.7719) ccw
  arc A197 (-117.4787, 33.1932) -> (-118.5393, 32.7539) centre (-117.4787, 31.6932) ccw
  line L188 (-43.9, 65.3932) -> (-43.9, 73.8932)
  line L189 (-28.9, 63.3932) -> (-41.9, 63.3932)
  line L190 (-60.9, 59.1932) -> (-48.3213, 59.1932)
  line L191 (-45.9, 56.7719) -> (-45.9, 48.6932)
  line L192 (-47.2607, 58.7539) -> (-46.3393, 57.8325)
  arc A198 (-47.2607, 58.7539) -> (-48.3213, 59.1932) centre (-48.3213, 57.6932) ccw
  arc A199 (-45.9, 56.7719) -> (-46.3393, 57.8325) centre (-47.4, 56.7719) ccw
  line L193 (-43.9, 27.3932) -> (-43.9, 35.8932)
  line L194 (-28.9, 25.3932) -> (-41.9, 25.3932)
  line L195 (-60.9, 21.1932) -> (-48.3213, 21.1932)
  line L196 (-45.9, 18.7719) -> (-45.9, 10.6932)
  line L197 (-47.2607, 20.7539) -> (-46.3393, 19.8325)
  arc A200 (-47.2607, 20.7539) -> (-48.3213, 21.1932) centre (-48.3213, 19.6932) ccw
  arc A201 (-45.9, 18.7719) -> (-46.3393, 19.8325) centre (-47.4, 18.7719) ccw
  line L198 (-138.1, 14.5932) -> (-103.1426, 14.5932)
  arc A202 (-103.1426, 14.5932) -> (-100.8799, 15.5305) centre (-103.1426, 17.7931) ccw
  line L199 (-100.8799, 15.5305) -> (-94.6373, 21.7731)
  arc A203 (-92.6574, 22.5932) -> (-94.6373, 21.7731) centre (-92.6573, 19.7931) ccw
  line L200 (-92.6574, 22.5932) -> (-76.2344, 22.5932)
  arc A204 (-72.9258, 20.6624) -> (-76.2344, 22.5932) centre (-76.2344, 18.793) ccw
  line L201 (-64.6482, 6.011) -> (-72.9258, 20.6624)
  arc A205 (-64.6482, 6.011) -> (-62.7328, 4.8932) centre (-62.7328, 7.0932) ccw
  line L202 (-48.0284, 4.8932) -> (-62.7328, 4.8932)
  arc A206 (-46.7556, 4.366) -> (-48.0284, 4.8932) centre (-48.0284, 3.0933) ccw
  line L203 (-45.6272, 3.2376) -> (-46.7556, 4.366)
  arc A207 (-45.6272, 3.2376) -> (-44.0716, 2.5932) centre (-44.0715, 4.7933) ccw
  line L204 (-44.0716, 2.5932) -> (-29.0284, 2.5932)
  arc A208 (-27.7556, 2.066) -> (-29.0284, 2.5932) centre (-29.0284, 0.7933) ccw
  line L205 (-26.6272, 0.9376) -> (-27.7556, 2.066)
  arc A209 (-26.6272, 0.9376) -> (-25.0716, 0.2932) centre (-25.0715, 2.4933) ccw
  line L206 (-8.6, 0.2932) -> (-25.0716, 0.2932)
  arc A210 (-8.6, 0.2932) -> (-6.9, 1.9932) centre (-8.6, 1.9932) ccw
  line L207 (-6.9, 1.9932) -> (-6.9, 76.4932)
  arc A211 (-6.9, 76.4932) -> (-8.6, 78.1932) centre (-8.6, 76.4932) ccw
  line L208 (-41.7716, 78.1932) -> (-8.6, 78.1932)
  arc A212 (-43.0444, 78.7204) -> (-41.7716, 78.1932) centre (-41.7716, 79.9932) ccw
  line L209 (-43.0444, 78.7204) -> (-44.1728, 79.8488)
  arc A213 (-44.1728, 79.8488) -> (-45.7284, 80.4932) centre (-45.7285, 78.2931) ccw
  line L210 (-58.5716, 80.4932) -> (-45.7284, 80.4932)
  arc A214 (-59.8444, 81.0204) -> (-58.5716, 80.4932) centre (-58.5716, 82.2931) ccw
  line L211 (-63.1728, 84.3488) -> (-59.8444, 81.0204)
  arc A215 (-63.1728, 84.3488) -> (-64.7284, 84.9932) centre (-64.7285, 82.7931) ccw
  line L212 (-82.0716, 84.9932) -> (-64.7284, 84.9932)
  arc A216 (-82.0716, 84.9932) -> (-83.6272, 84.3488) centre (-82.0716, 82.7933) ccw
  line L213 (-83.6272, 84.3488) -> (-85.9556, 82.0204)
  arc A217 (-87.2284, 81.4932) -> (-85.9556, 82.0204) centre (-87.2284, 83.2932) ccw
  line L214 (-101.0716, 81.4932) -> (-87.2284, 81.4932)
  arc A218 (-101.0716, 81.4932) -> (-102.6272, 80.8488) centre (-101.0716, 79.2933) ccw
  line L215 (-102.6272, 80.8488) -> (-109.1627, 74.3133)
  arc A219 (-111.1426, 73.4932) -> (-109.1627, 74.3133) centre (-111.1426, 76.2932) ccw
  line L216 (-120.0716, 73.4932) -> (-111.1426, 73.4932)
  arc A220 (-120.0716, 73.4932) -> (-121.6272, 72.8488) centre (-120.0716, 71.2933) ccw
  line L217 (-122.7556, 71.7204) -> (-121.6272, 72.8488)
  arc A221 (-124.0284, 71.1932) -> (-122.7556, 71.7204) centre (-124.0284, 72.9932) ccw
  line L218 (-138.1, 71.1932) -> (-124.0284, 71.1932)
  arc A222 (-138.1, 71.1932) -> (-139.8, 69.4932) centre (-138.1, 69.4932) ccw
  line L219 (-139.8, 69.4932) -> (-139.8, 16.2932)
  arc A223 (-139.8, 16.2932) -> (-138.1, 14.5932) centre (-138.1, 16.2932) ccw
  line L220 (-82.7757, 87.4932) -> (-64.0243, 87.4932)
  line L221 (-84.8971, 86.6145) -> (-87.2255, 84.2861)
  line L222 (-101.7757, 83.9932) -> (-87.9326, 83.9932)
  line L223 (-103.8971, 83.1145) -> (-110.579, 76.4325)
  line L224 (-120.7757, 75.9932) -> (-111.6397, 75.9932)
  line L225 (-124.0255, 73.9861) -> (-122.8971, 75.1145)
  line L226 (-138.3, 73.6932) -> (-124.7326, 73.6932)
  line L227 (-142.3, 69.6932) -> (-142.3, 16.0932)
  line L228 (-138.3, 12.0932) -> (-102.6456, 12.0932)
  line L229 (-99.4636, 13.4112) -> (-93.3674, 19.5074)
  line L230 (-91.9532, 20.0932) -> (-77.2264, 20.0932)
  line L231 (-66.4804, 4.1716) -> (-74.6144, 18.5689)
  line L232 (-48.7326, 2.3932) -> (-63.4331, 2.3932)
  line L233 (-44.7757, 0.0932) -> (-29.7326, 0.0932)
  line L234 (-8.4, -2.2068) -> (-25.7757, -2.2068)
  line L235 (-4.4, 1.7932) -> (-4.4, 76.6932)
  line L236 (-41.0674, 80.6932) -> (-8.4, 80.6932)
  line L237 (-41.7745, 80.9861) -> (-42.9029, 82.1145)
  line L238 (-57.8674, 82.9932) -> (-45.0243, 82.9932)
  line L239 (-61.9029, 86.6145) -> (-58.5745, 83.2861)
  line L240 (-27.8971, -1.3281) -> (-29.0255, -0.1997)
  line L241 (-46.8971, 0.9719) -> (-48.0255, 2.1003)
  arc A224 (-138.3, 73.6932) -> (-142.3, 69.6932) centre (-138.3, 69.6932) ccw
  arc A225 (-142.3, 16.0932) -> (-138.3, 12.0932) centre (-138.3, 16.0932) ccw
  arc A226 (-4.4, 76.6932) -> (-8.4, 80.6932) centre (-8.4, 76.6932) ccw
  arc A227 (-8.4, -2.2068) -> (-4.4, 1.7932) centre (-8.4, 1.7932) ccw
  arc A228 (-124.7326, 73.6932) -> (-124.0255, 73.9861) centre (-124.7326, 74.6932) ccw
  arc A229 (-120.7757, 75.9932) -> (-122.8971, 75.1145) centre (-120.7757, 72.9932) ccw
  arc A230 (-111.6397, 75.9932) -> (-110.579, 76.4325) centre (-111.6397, 77.4932) ccw
  arc A231 (-101.7757, 83.9932) -> (-103.8971, 83.1145) centre (-101.7757, 80.9932) ccw
  arc A232 (-87.9326, 83.9932) -> (-87.2255, 84.2861) centre (-87.9326, 84.9932) ccw
  arc A233 (-82.7757, 87.4932) -> (-84.8971, 86.6145) centre (-82.7757, 84.4932) ccw
  arc A234 (-61.9029, 86.6145) -> (-64.0243, 87.4932) centre (-64.0243, 84.4932) ccw
  arc A235 (-58.5745, 83.2861) -> (-57.8674, 82.9932) centre (-57.8674, 83.9932) ccw
  arc A236 (-42.9029, 82.1145) -> (-45.0243, 82.9932) centre (-45.0243, 79.9932) ccw
  arc A237 (-41.7745, 80.9861) -> (-41.0674, 80.6932) centre (-41.0674, 81.6932) ccw
  arc A238 (-27.8971, -1.3281) -> (-25.7757, -2.2068) centre (-25.7757, 0.7932) ccw
  arc A239 (-29.0255, -0.1997) -> (-29.7326, 0.0932) centre (-29.7326, -0.9068) ccw
  arc A240 (-46.8971, 0.9719) -> (-44.7757, 0.0932) centre (-44.7757, 3.0932) ccw
  arc A241 (-48.0255, 2.1003) -> (-48.7326, 2.3932) centre (-48.7326, 1.3932) ccw
  arc A242 (-66.4804, 4.1716) -> (-63.4331, 2.3932) centre (-63.4331, 5.8932) ccw
  arc A243 (-74.6144, 18.5689) -> (-77.2264, 20.0932) centre (-77.2264, 17.0932) ccw
  arc A244 (-91.9532, 20.0932) -> (-93.3674, 19.5074) centre (-91.9532, 18.0932) ccw
  arc A245 (-102.6456, 12.0932) -> (-99.4636, 13.4112) centre (-102.6456, 16.5932) ccw
  line L242 (-7.5, 12.9932) -> (-7.5, 6.1932)
  line L243 (-25, 22.0932) -> (-25, 73.8932)
  circle A246 centre (-44.9, 22.5432) radius 1.15
  circle A247 centre (-44.9, 60.5432) radius 1.15
  circle A248 centre (-120.9, 53.5432) radius 1.15
  circle A249 centre (-120.9, 34.5432) radius 1.15
  line L244 (-20.5, 77.5932) -> (-8.6, 77.5932)
  line L245 (-7.4999, 40.5932) -> (-7.5, 76.4932)
  arc A250 (-7.5, 76.4932) -> (-8.6, 77.5932) centre (-8.6, 76.4932) ccw
  arc A251 (-21.1, 78.1932) -> (-20.5, 77.5932) centre (-20.5, 78.1932) ccw
  arc A252 (-7.5, 6.1932) -> (-6.9, 5.5932) centre (-6.9, 6.1932) ccw
  arc A253 (-123.9, 56.3932) -> (-121.9, 58.3932) centre (-123.9, 58.3932) ccw
  arc A254 (-123.9, 37.3932) -> (-121.9, 39.3932) centre (-123.9, 39.3932) ccw
  arc A255 (-43.9, 65.3932) -> (-41.9, 63.3932) centre (-41.9, 65.3932) ccw
  arc A256 (-43.9, 27.3932) -> (-41.9, 25.3932) centre (-41.9, 27.3932) ccw
  line L246 (-6.8999, 39.9932) -> (-6.9, 39.9932)
  arc A257 (-7.4999, 40.5932) -> (-6.8999, 39.9932) centre (-6.8999, 40.5932) ccw
  line L247 (-23, 75.8932) -> (-9.7, 75.8932)
  arc A258 (-15.1, 20.7932) -> (-15.1, 24.1932) centre (-15.1, 22.4932) ccw construction
  arc A259 (-17.7, 24.1932) -> (-17.7, 20.7932) centre (-17.7, 22.4932) ccw construction
  line L248 (-17.7, 24.1932) -> (-15.1, 24.1932) construction
  line L249 (-15.1, 20.7932) -> (-17.7, 20.7932) construction
  line L250 (-25, 72.0932) -> (-7.7, 72.0932)
  line L251 (-23, 20.0932) -> (-9.7, 20.0932)
  arc A260 (-6.9, 13.5932) -> (-7.5, 12.9932) centre (-6.9, 12.9932) ccw
  line L252 (-7.7, 73.8932) -> (-7.7, 22.0932)
  arc A261 (-25, 22.0932) -> (-23, 20.0932) centre (-23, 22.0932) ccw
  arc A262 (-9.7, 20.0932) -> (-7.7, 22.0932) centre (-9.7, 22.0932) ccw
  arc A263 (-23, 75.8932) -> (-25, 73.8932) centre (-23, 73.8932) ccw
  arc A264 (-7.7, 73.8932) -> (-9.7, 75.8932) centre (-9.7, 73.8932) ccw
  line L253 (-25, 24.8932) -> (-7.7, 24.8932)
  point P0 (19.2932, 12.1)
  dimension "d1" = 3.4
  dimension "d2" = 3.4
  dimension "d3" = 8
  dimension "d4" = 3.4
  dimension "d5" = 3.4
  dimension "d9" = 2.3
  dimension "d12" = 2.3
  dimension "d367" = 2.3
  dimension "d368" = 2.3
  dimension "d369" = 2.3
  dimension "d370" = 2.3
  constraint tangent L19 A5
  constraint tangent L19 A6
  constraint tangent L13 A7
  constraint tangent L17 A8
  constraint tangent L12 A9
  constraint tangent L16 A10
  constraint tangent L8 A11
  constraint tangent L7 A13
  constraint tangent L9 A14
  constraint tangent L18 A15
  constraint tangent L2 A16
  constraint tangent L0 A17
  constraint tangent L10 A18
  constraint tangent L5 A19
  constraint tangent L11 A20
  constraint tangent L6 A21
  constraint tangent L3 A22
  constraint tangent L1 A23
  constraint tangent L4 A24
  constraint tangent L15 A25
  constraint tangent A24 L104
  constraint perpendicular L104 L105
  constraint tangent L104 A26
  constraint tangent L105 A26
  constraint coincident L15.end L105
  constraint perpendicular L15 L105
  constraint coincident L14.end L104
  constraint perpendicular L14 L104
  constraint tangent L32 A27
  constraint tangent L33 A28
  constraint tangent L35 A29
  constraint tangent L34 A30
  constraint tangent L49 A31
  constraint tangent L49 A32
  constraint tangent L51 A33
  constraint tangent L50 A34
  constraint tangent L57 A35
  constraint tangent L57 A36
  constraint tangent L59 A37
  constraint tangent L58 A38
  constraint tangent L76 A39
  constraint tangent L78 A40
  constraint tangent L79 A41
  constraint tangent L77 A42
  constraint tangent L54 A43
  constraint tangent L54 A44
  constraint tangent L52 A45
  constraint tangent L53 A46
  constraint tangent L90 A47
  constraint tangent L90 A48
  constraint tangent L91 A48
  constraint tangent L91 A49
  constraint tangent L89 A50
  constraint tangent L100 A51
  constraint tangent L101 A52
  constraint tangent L103 A53
  constraint tangent L102 A54
  constraint tangent L93 A55
  constraint tangent L93 A56
  constraint tangent L95 A57
  constraint tangent L94 A58
  constraint tangent L21 A59
  constraint tangent L20 A60
  constraint tangent L22 A60
  constraint tangent L22 A61
  constraint tangent L23 A62
  constraint tangent L64 A63
  constraint tangent L66 A63
  constraint tangent L64 A64
  constraint tangent L65 A65
  constraint tangent L67 A66
  constraint tangent L98 A67
  constraint tangent L98 A68
  constraint tangent L96 A69
  constraint tangent L97 A70
  constraint tangent L70 A71
  constraint tangent L70 A72
  constraint tangent L68 A73
  constraint tangent L69 A74
  constraint tangent L80 A75
  constraint tangent L80 A76
  constraint tangent L82 A76
  constraint tangent L82 A77
  constraint tangent L83 A77
  constraint tangent L83 A78
  constraint tangent L81 A78
  constraint tangent L29 A79
  constraint tangent L29 A80
  constraint tangent L28 A81
  constraint tangent L30 A82
  constraint tangent L37 A83
  constraint tangent L37 A84
  constraint tangent L36 A84
  constraint tangent L36 A85
  constraint tangent L38 A85
  constraint tangent L38 A86
  constraint tangent L39 A86
  constraint tangent L61 A87
  constraint tangent L61 A88
  constraint tangent L60 A88
  constraint tangent L60 A89
  constraint tangent L62 A90
  constraint tangent L40 A91
  constraint tangent L42 A92
  constraint tangent L43 A93
  constraint tangent L41 A93
  constraint tangent L41 A94
  constraint tangent L40 A94
  constraint tangent L44 A95
  constraint tangent L46 A95
  constraint tangent L46 A96
  constraint tangent L47 A96
  constraint tangent L47 A97
  constraint tangent L45 A97
  constraint tangent L45 A98
  constraint tangent L44 A98
  constraint tangent L74 A99
  constraint tangent L75 A99
  constraint tangent L74 A100
  constraint tangent L72 A101
  constraint tangent L73 A102
  constraint tangent L26 A103
  constraint tangent L27 A103
  constraint tangent L26 A104
  constraint tangent L24 A105
  constraint tangent L25 A106
  constraint tangent L86 A107
  constraint tangent L87 A107
  constraint tangent L86 A108
  constraint tangent L84 A109
  constraint tangent L85 A110
  constraint tangent A12 L107
  constraint tangent L106 A113
  constraint tangent L107 A113
  constraint concentric A8 A114
  constraint concentric A6 A115
  constraint concentric A23 A116
  constraint concentric A21 A117
  constraint parallel L108 L183
  constraint tangent A118 L183
  constraint tangent L109 A118
  constraint tangent L108 A119
  constraint tangent L108 A120
  constraint tangent L109 A120
  constraint parallel L110 L178
  constraint tangent A123 L178
  constraint tangent L111 A123
  constraint tangent A121 L110
  constraint tangent L110 A122
  constraint tangent A122 L111
  constraint horizontal L112
  constraint perpendicular L112 L113
  constraint parallel L112 L114
  constraint parallel L113 L115
  constraint tangent A127 L115
  constraint tangent L114 A127
  constraint tangent A124 L112
  constraint tangent A124 L115
  constraint tangent L112 A125
  constraint tangent A125 L113
  constraint tangent L113 A126
  constraint tangent A126 L114
  constraint horizontal L116
  constraint perpendicular L116 L117
  constraint parallel L116 L118
  constraint parallel L117 L119
  constraint tangent A131 L119
  constraint tangent L118 A131
  constraint tangent A128 L116
  constraint tangent A128 L119
  constraint tangent L116 A129
  constraint tangent A129 L117
  constraint tangent L117 A130
  constraint tangent A130 L118
  constraint horizontal L120
  constraint perpendicular L120 L186
  constraint parallel L121 L186
  constraint tangent A134 L121
  constraint tangent A132 L120
  constraint tangent A132 L121
  constraint tangent L120 A133
  constraint tangent A133 L186
  constraint horizontal L122
  constraint perpendicular L122 L181
  constraint parallel L123 L181
  constraint tangent A137 L123
  constraint tangent A135 L122
  constraint tangent A135 L123
  constraint tangent L122 A136
  constraint tangent A136 L181
  constraint horizontal L124
  constraint perpendicular L124 L125
  constraint parallel L124 L126
  constraint parallel L125 L127
  constraint tangent A141 L127
  constraint tangent L126 A141
  constraint tangent A138 L124
  constraint tangent A138 L127
  constraint tangent L124 A139
  constraint tangent A139 L125
  constraint tangent L125 A140
  constraint tangent A140 L126
  constraint horizontal L128
  constraint perpendicular L128 L129
  constraint parallel L128 L130
  constraint parallel L129 L131
  constraint tangent A145 L131
  constraint tangent L130 A145
  constraint tangent A142 L128
  constraint tangent A142 L131
  constraint tangent L128 A143
  constraint tangent A143 L129
  constraint tangent L129 A144
  constraint tangent A144 L130
  constraint horizontal L132
  constraint perpendicular L132 L133
  constraint parallel L132 L134
  constraint parallel L133 L135
  constraint tangent A149 L135
  constraint tangent L134 A149
  constraint tangent A146 L132
  constraint tangent A146 L135
  constraint tangent L132 A147
  constraint tangent A147 L133
  constraint tangent L133 A148
  constraint tangent A148 L134
  constraint horizontal L144
  constraint perpendicular L144 L145
  constraint parallel L144 L146
  constraint parallel L145 L147
  constraint tangent A161 L147
  constraint tangent L146 A161
  constraint tangent A158 L144
  constraint tangent A158 L147
  constraint tangent L144 A159
  constraint tangent A159 L145
  constraint tangent L145 A160
  constraint tangent A160 L146
  constraint horizontal L140
  constraint perpendicular L140 L141
  constraint parallel L140 L142
  constraint parallel L141 L143
  constraint tangent A157 L143
  constraint tangent L142 A157
  constraint tangent A154 L140
  constraint tangent A154 L143
  constraint tangent L140 A155
  constraint tangent A155 L141
  constraint tangent L141 A156
  constraint tangent A156 L142
  constraint horizontal L136
  constraint perpendicular L136 L137
  constraint parallel L136 L138
  constraint parallel L137 L139
  constraint tangent A153 L139
  constraint tangent L138 A153
  constraint tangent A150 L136
  constraint tangent A150 L139
  constraint tangent L136 A151
  constraint tangent A151 L137
  constraint tangent L137 A152
  constraint tangent A152 L138
  constraint horizontal L154
  constraint perpendicular L154 L155
  constraint parallel L154 L156
  constraint parallel L155 L157
  constraint tangent A172 L157
  constraint tangent L156 A172
  constraint tangent A169 L154
  constraint tangent A169 L157
  constraint tangent L154 A170
  constraint tangent A170 L155
  constraint tangent L155 A171
  constraint tangent A171 L156
  constraint horizontal L152
  constraint perpendicular L152 L153
  constraint parallel L152 L190
  constraint tangent A166 L152
  constraint tangent L152 A167
  constraint tangent A167 L153
  constraint tangent L153 A168
  constraint tangent A168 L190
  constraint horizontal L148
  constraint perpendicular L148 L149
  constraint parallel L148 L150
  constraint parallel L149 L151
  constraint tangent A165 L151
  constraint tangent L150 A165
  constraint tangent A162 L148
  constraint tangent A162 L151
  constraint tangent L148 A163
  constraint tangent A163 L149
  constraint tangent L149 A164
  constraint tangent A164 L150
  constraint horizontal L158
  constraint perpendicular L158 L159
  constraint parallel L158 L195
  constraint tangent A173 L158
  constraint tangent L158 A174
  constraint tangent A174 L159
  constraint tangent L159 A175
  constraint tangent A175 L195
  constraint horizontal L189
  constraint parallel L170 L189
  constraint tangent A189 L171
  constraint tangent L170 A189
  constraint tangent A187 L189
  constraint tangent A187 L171
  constraint tangent A188 L170
  constraint horizontal L166
  constraint perpendicular L166 L167
  constraint parallel L166 L168
  constraint parallel L167 L169
  constraint tangent A186 L169
  constraint tangent L168 A186
  constraint tangent A183 L166
  constraint tangent A183 L169
  constraint tangent L166 A184
  constraint tangent A184 L167
  constraint tangent L167 A185
  constraint tangent A185 L168
  constraint horizontal L194
  constraint parallel L164 L194
  constraint tangent A182 L165
  constraint tangent L164 A182
  constraint tangent A180 L194
  constraint tangent A180 L165
  constraint tangent A181 L164
  constraint horizontal L160
  constraint perpendicular L160 L161
  constraint parallel L160 L162
  constraint parallel L161 L163
  constraint tangent A179 L163
  constraint tangent L162 A179
  constraint tangent A176 L160
  constraint tangent A176 L163
  constraint tangent L160 A177
  constraint tangent A177 L161
  constraint tangent L161 A178
  constraint tangent A178 L162
  constraint horizontal L172
  constraint perpendicular L172 L173
  constraint parallel L172 L174
  constraint parallel L173 L175
  constraint tangent A193 L175
  constraint tangent L174 A193
  constraint tangent A190 L172
  constraint tangent A190 L175
  constraint tangent L172 A191
  constraint tangent A191 L173
  constraint tangent L173 A192
  constraint tangent A192 L174
  constraint tangent L185 A194
  constraint tangent L187 A194
  constraint tangent L186 A195
  constraint tangent L187 A195
  constraint tangent L181 A196
  constraint tangent L182 A196
  constraint tangent L180 A197
  constraint tangent L182 A197
  constraint tangent L190 A198
  constraint tangent L192 A198
  constraint tangent L191 A199
  constraint tangent L192 A199
  constraint tangent L195 A200
  constraint tangent L197 A200
  constraint tangent L196 A201
  constraint tangent L197 A201
  constraint coincident L208 L176.start
  constraint coincident L207 L177.start
  constraint coincident L236 L176.end
  constraint coincident L235 L177.end
  constraint tangent L226 A224
  constraint tangent L227 A224
  constraint tangent L227 A225
  constraint tangent L228 A225
  constraint tangent L236 A226
  constraint tangent L235 A226
  constraint tangent L235 A227
  constraint tangent L234 A227
  constraint tangent L225 A228
  constraint tangent L226 A228
  constraint tangent L224 A229
  constraint tangent L225 A229
  constraint tangent L223 A230
  constraint tangent L224 A230
  constraint tangent L222 A231
  constraint tangent L223 A231
  constraint tangent L221 A232
  constraint tangent L222 A232
  constraint tangent L220 A233
  constraint tangent L221 A233
  constraint tangent L220 A234
  constraint tangent L239 A234
  constraint tangent L238 A235
  constraint tangent L239 A235
  constraint tangent L238 A236
  constraint tangent L237 A236
  constraint tangent L236 A237
  constraint tangent L237 A237
  constraint tangent L240 A238
  constraint tangent L234 A238
  constraint tangent L233 A239
  constraint tangent L240 A239
  constraint tangent L241 A240
  constraint tangent L233 A240
  constraint tangent L232 A241
  constraint tangent L241 A241
  constraint tangent L232 A242
  constraint tangent L231 A242
  constraint tangent L231 A243
  constraint tangent L230 A243
  constraint tangent L230 A244
  constraint tangent L229 A244
  constraint tangent L229 A245
  constraint tangent L228 A245
  constraint concentric A3 A246
  constraint concentric A4 A247
  constraint concentric A0 A248
  constraint concentric A1 A249
  constraint vertical L242
  constraint tangent L244 A250
  constraint tangent L245 A250
  constraint tangent L244 A251
  constraint tangent L242 A252
  constraint tangent L183 A253
  constraint tangent L184 A253
  constraint tangent L178 A254
  constraint tangent L179 A254
  constraint tangent L189 A255
  constraint tangent L188 A255
  constraint tangent L193 A256
  constraint tangent L194 A256
  constraint perpendicular L207 L246
  constraint coincident L207 L246.end
  constraint tangent L246 A257